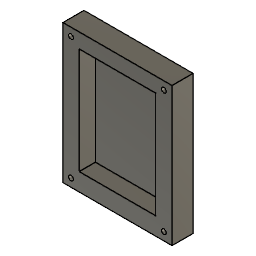
new_back_case (Autodesk Fusion 360 design; units mm, degrees)
part number: 2026-02-06-21-37-17-528
Autodesk Fusion 360 part; units mm, degrees
sketch "Sketch1" plane through (0, 0, 0) normal (0, 1, 0) x (1, 0, 0)
  line L0 (-48.8546, -55.3051) -> (-1.7146, -55.3051)
  line L1 (-1.7146, -55.3051) -> (-1.7146, 10.0349)
  line L2 (-1.7146, 10.0349) -> (-48.8546, 10.0349)
  line L3 (-48.8546, 10.0349) -> (-48.8546, -55.3051)
  line L4 (-58.8546, -65.3051) -> (8.2854, -65.3051)
  line L5 (8.2854, -65.3051) -> (8.2854, 20.0349)
  line L6 (8.2854, 20.0349) -> (-58.8546, 20.0349)
  line L7 (-58.8546, 20.0349) -> (-58.8546, -65.3051)
  circle A0 centre (-53.8546, -60.3051) radius 1.45
  circle A1 centre (-53.8546, 15.0349) radius 1.45
  circle A2 centre (3.2854, 15.0349) radius 1.45
  circle A3 centre (3.2854, -60.3051) radius 1.45
  dimension "d1" = 47.14
  dimension "d2" = 65.34
  dimension "d3" = 10
  dimension "d4" = 10
  dimension "d5" = 10
  dimension "d6" = 10
  dimension "d7" = 2.9
  dimension "d8" = 5
  dimension "d9" = 5
  dimension "d10" = 2.9
  dimension "d11" = 5
  dimension "d12" = 5
  dimension "d13" = 2.9
  dimension "d14" = 5
  dimension "d15" = 5
  dimension "d16" = 2.9
  dimension "d17" = 5
  dimension "d18" = 5
  constraint horizontal L0
  constraint vertical L1
  constraint horizontal L2
  constraint vertical L3
  constraint horizontal L4
  constraint vertical L5
  constraint horizontal L6
  constraint vertical L7
  measures "d1" distance of L0.start L0.end
  measures "d2" distance of L0 L2
  measures "d3" distance of L0 L4
  measures "d4" distance of L1 L5
  measures "d5" distance of L2 L6
  measures "d6" distance of L3 L7
  measures "d7" diameter of A0
  measures "d8" distance of L4 A0.centre
  measures "d9" distance of L7 A0.centre
  measures "d10" diameter of A1
  measures "d11" distance of L6 A1.centre
  measures "d12" distance of L7 A1.centre
  measures "d13" diameter of A2
  measures "d14" distance of L5 A2.centre
  measures "d15" distance of L6 A2.centre
  measures "d16" diameter of A3
  measures "d17" distance of L5 A3.centre
  measures "d18" distance of L4 A3.centre
extrude "Extrude1" add sketch "Sketch1" along normal blind 10 contours L0 L1 L2 L3 | L4 L5 L6 L7
sketch "Sketch2" plane through (0, 0, 0) normal (0, 1, 0) x (1, 0, 0)
  line L0 (-48.8399, -56.2293) -> (-1.6999, -56.2293)
  line L1 (-1.6999, -56.2293) -> (-1.6999, 9.1107)
  line L2 (-1.6999, 9.1107) -> (-48.8399, 9.1107)
  line L3 (-48.8399, 9.1107) -> (-48.8399, -56.2293)
  dimension "d21" = 47.14
  dimension "d22" = 65.34
  constraint horizontal L0
  constraint vertical L1
  constraint horizontal L2
  constraint vertical L3
  measures "d21" distance of L0.start L0.end
  measures "d22" distance of L0 L2
extrude "Extrude2" cut sketch "Sketch2" along normal blind 7
extrude "Extrude3" add 1 faces at (-33.1363, 0, -13.4796) along direction (0, -1, 0) blind 3
